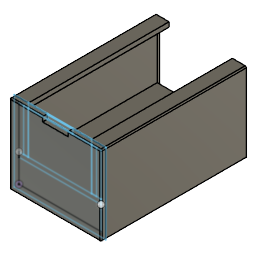
TA-boitier-V1 (Autodesk Fusion 360 design; units mm, degrees)
part number: 2025-12-22-10-16-26-791
Autodesk Fusion 360 part; units mm, degrees
sketch "Esquisse1" plane through (0, 0, 0) normal (0, 1, 0) x (1, 0, 0)
  line L0 (0, 0) -> (35, 0)
  line L1 (35, 0) -> (35, -10)
  line L2 (0, -10) -> (0, 0)
  line L3 (35, -10) -> (35, -30.0216)
  line L4 (35, -30.0216) -> (0, -30.0216)
  line L5 (0, -30.0216) -> (0, -10)
  line L6 (4, -30.0216) -> (4, -12.0216)
  line L7 (31, -30.0216) -> (31, -12.0794)
  line L8 (23, -32.0216) -> (12.0758, -32.0216)
  line L9 (12.0758, -32.0216) -> (12.0758, -30.0216)
  line L10 (12.0758, -30.0216) -> (23, -30.0216)
  line L11 (23, -30.0216) -> (23, -32.0216)
  line L12 (-2, -32.0216) -> (37, -32.0216)
  line L13 (37, -32.0216) -> (37, 2)
  line L14 (37, 2) -> (-2, 2)
  line L15 (-2, 2) -> (-2, -32.0216)
  line L16 (2, -30) -> (4, -30)
  line L17 (4, -30) -> (4, -12.0216)
  line L18 (4, -12.0216) -> (2, -12.0216)
  line L19 (2, -12.0216) -> (2, -30)
  line L20 (33.0971, -30.0216) -> (31, -30.0216)
  line L21 (31, -30.0216) -> (31, -12.0794)
  line L22 (31, -12.0794) -> (33.0971, -12.0794)
  line L23 (33.0971, -12.0794) -> (33.0971, -30.0216)
  line L24 (35, -10) -> (35, -12)
  line L25 (0, -12) -> (0, -10)
  line L26 (35, -12) -> (0, -12)
  line L27 (0, -12) -> (0, -10)
  line L28 (0, -10) -> (35, -10)
  line L29 (35, -10) -> (35, -12)
  line L30 (4.0433, -32.0216) -> (31, -32.0216)
  line L31 (31, -32.0216) -> (31, -30.0216)
  line L32 (31, -30.0216) -> (4.0433, -30.0216)
  line L33 (4.0433, -30.0216) -> (4.0433, -32.0216)
  constraint horizontal L0
  constraint vertical L1
  constraint vertical L2
  constraint coincident L0.start L2.end
  constraint vertical L3
  constraint horizontal L4
  constraint vertical L5
  constraint coincident L4 L6.start
  constraint coincident L4 L7.start
  constraint horizontal L8
  constraint vertical L9
  constraint horizontal L10
  constraint vertical L11
  constraint horizontal L12
  constraint vertical L13
  constraint horizontal L14
  constraint vertical L15
  constraint horizontal L16
  constraint vertical L17
  constraint horizontal L18
  constraint vertical L19
  constraint horizontal L20
  constraint vertical L21
  constraint horizontal L22
  constraint vertical L23
  constraint coincident L4 L20.start
  constraint vertical L24
  constraint vertical L25
  constraint coincident L3 L24.end
  constraint horizontal L26
  constraint vertical L27
  constraint horizontal L28
  constraint vertical L29
  constraint horizontal L30
  constraint vertical L31
  constraint horizontal L32
  constraint vertical L33
  constraint coincident L12 L30.start
extrude "Extrusion2" add sketch "Esquisse1" against normal blind 2 contours L0 L1 L2 L3 L4 L5 L12 L13 L14 L15 L20 L24 L25 L27 L29 L31 L33 | L0 L1 L2 L28 | L3 L5 L24 L25 L26 L27 L28 L29 | L3 L4 L5 L7 L10 L21 L22 L23 L26 L32 | L4 L7 L20 L21 L22 L23 | L4 L9 L12 L30 L32 L33 | L4 L11 L12 L30 L31 L32 | L6 L16 L17 L18 L19 makes body 1
extrude "Extrusion3" add sketch "Esquisse1" along normal blind 60 separate body contours L0 L1 L2 L3 L4 L5 L12 L13 L14 L15 L20 L24 L25 L27 L29 L31 L33 makes body 2
extrude "Extrusion4" add sketch "Esquisse1" along normal blind 55 contours L3 L5 L24 L25 L26 L27 L28 L29 | L4 L7 L20 L21 L22 L23 | L6 L16 L17 L18 L19 bodies 2 makes body 3 at (2, 18.3333, 18.0144)
fillet "Congé1" radius 0.5 4 edges at (-2, -1, 32.0216) (37, -1, 32.0216) (-2, 30, 32.0216) (37, 30, 32.0216) on bodies 1 2
fillet "Congé2" radius 0.5 11 edges at (5.2879, -2, 32.0216) (-1.8536, -2, 31.8752) (-2, -2, 14.7608) (37, -2, 14.7608) (36.8536, -2, 31.8752) (29.75, -2, 32.0216) (-2, -1, -2) (17.5, -2, -2) (37, -1, -2) (-2, 30, -2) (37, 30, -2) on bodies 1 2
